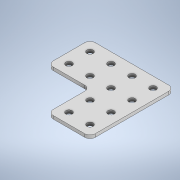
# Autodesk Inventor part: RightAngle_4040
Saved by Autodesk Inventor 2021 (Build 250183000, 183)
## iProperties
Created: 2022-01-07
Part Number: RightAngle_4040
Material: Generic
Document SubType Name: Modeling
Designer: Jorian Brusind
Density: 1 g/cm^3
Appearance: Default
Author: Jorian Brusind
Autodesk Inventor part; units mm, degrees
ref_plane "YZ Plane" through (0, 0, 0) normal (1, 0, 0) x (0, 1, 0)
ref_plane "XZ Plane" through (0, 0, 0) normal (0, 1, 0) x (-1, 0, 0)
ref_plane "XY Plane" through (0, 0, 0) normal (0, 0, 1) x (1, 0, 0)
sketch "Sketch1" plane through (0, 0, 0) normal (0, 1, 0) x (-1, 0, 0)
  line L0 (0, 0) -> (40, 0)
  line L1 (40, 0) -> (40, -80)
  line L2 (40, -80) -> (0, -80)
  line L3 (0, -80) -> (0, 0)
  line L4 (0, -80) -> (80, -80)
  line L5 (80, -80) -> (80, -40)
  line L6 (80, -40) -> (0, -40)
  line L7 (0, -40) -> (0, -80)
  point P0 (40, -40)
  dimension "d0" = 40
  dimension "d1" = 80
  dimension "d2" = 80
  dimension "d3" = 40
  constraints: 16 end point, 4 parallel, 2 horizontal, 2 perpendicular
  measures "d0" distance of L1.end L2.end
  measures "d1" distance of L0.end L1.end
  measures "d2" distance of L6.end L5.end
  measures "d3" distance of L5.end L4.end
extrude "Extrusion1" add sketch "Sketch1" along normal blind 3
sketch "Sketch2" plane through (0, 3, 0) normal (0, 1, 0) x (1, 0, 0)
  line L0 (0, 0) -> (-10, 0)
  line L1 (-40, 0) -> (0, 0) projected
  line L2 (-10, 0) -> (-10, 10)
  circle A0 centre (-10, 10) radius 3
  line L3 (0, 0) -> (0, 80) projected
  line L4 (0, 0) -> (0, 80)
  circle A1 centre (-10, 30) radius 3
  circle A2 centre (-10, 50) radius 3
  circle A3 centre (-10, 70) radius 3
  circle A4 centre (-30, 10) radius 3
  circle A5 centre (-30, 30) radius 3
  circle A6 centre (-30, 50) radius 3
  circle A7 centre (-30, 70) radius 3
  line L5 (-10, 70) -> (0, 70)
  line L6 (-10, 70) -> (-10, 80)
  line L7 (0, 80) -> (-80, 80) projected
  circle A8 centre (-10, 70) radius 3
  circle A9 centre (-30, 70) radius 3
  circle A10 centre (-50, 70) radius 3
  circle A11 centre (-70, 70) radius 3
  circle A12 centre (-10, 50) radius 3
  circle A13 centre (-30, 50) radius 3
  circle A14 centre (-50, 50) radius 3
  circle A15 centre (-70, 50) radius 3
  dimension "d6" = 10
  dimension "d7" = 10
  dimension "d8" = 6
  dimension "d11" = 20
  dimension "d14" = 20
  dimension "d19" = 20
  dimension "d22" = 20
  constraints: 16 centre point, 10 end point, 3 perpendicular, 3 point on line, 3 vertical, 2 coincident, 2 horizontal, 28 other
  measures "d6" distance of L0.start L0.end
  measures "d7" distance of L0.end L2.end
  measures "d8" diameter of A0
  measures "d11" distance of A0.centre A1.centre
  measures "d14" distance of A0.centre A4.centre
  measures "d19" distance of L5.start A9.centre
  measures "d22" distance of L5.start A12.centre
extrude "Extrusion2" cut sketch "Sketch2" against normal through all contours A0 | L5 L6 A3 | A3 L6 L5 | A1 | A2 | A4 | A5 | A6 | A7 | A10 | A11 | A14 | A15
fillet "Fillet1" radius 5 6 edges at (0, 1.5, 0) (-40, 1.5, 0) (0, 1.5, -80) (-40, 1.5, -40) (-80, 1.5, -40) (-80, 1.5, -80)
body "Solid1"
